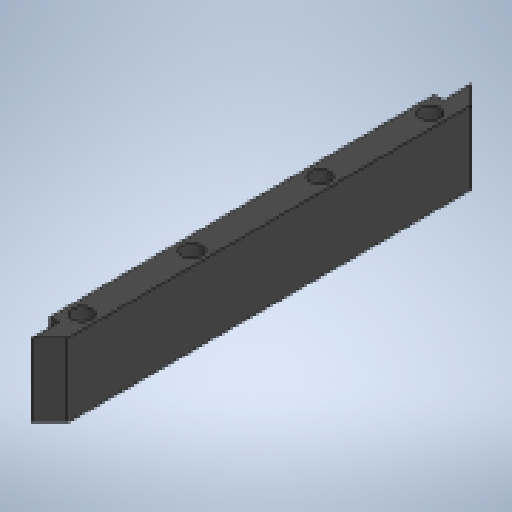
# Autodesk Inventor part: Backplate
Saved by Autodesk Inventor 2023.2 (Build 272271000, 271)
## iProperties
Created: 2023-06-29
Part Number: Backplate
Material: UHMW, Black
Document SubType Name: Modeling
Designer: Nathan Cai
Density: 0.94 g/cm^3
Appearance: Rubber - Black
Author: Nathan Cai
Autodesk Inventor part; units mm, degrees
ref_plane "YZ Plane" through (0, 0, 0) normal (1, 0, 0) x (0, 1, 0)
ref_plane "XZ Plane" through (0, 0, 0) normal (0, 1, 0) x (-1, 0, 0)
ref_plane "XY Plane" through (0, 0, 0) normal (0, 0, 1) x (1, 0, 0)
sketch "Sketch1" plane through (0, 0, 0) normal (0, 1, 0) x (-1, 0, 0)
  line L0 (-4.7625, 66.675) -> (4.7625, 66.675)
  line L1 (4.7625, 66.675) -> (4.7625, -66.675)
  line L2 (4.7625, -66.675) -> (-4.7625, -66.675)
  line L3 (-4.7625, -66.675) -> (-4.7625, 66.675)
  line L4 (-4.7625, 66.675) -> (4.7625, -66.675) construction
  line L5 (4.7625, 66.675) -> (-4.7625, -66.675) construction
  line L6 (-4.7625, 66.675) -> (1.5875, 66.675)
  line L7 (1.5875, 66.675) -> (1.5875, 76.2)
  line L8 (1.5875, 76.2) -> (-4.7625, 76.2)
  line L9 (-4.7625, 76.2) -> (-4.7625, 66.675)
  line L10 (4.7625, 0) -> (-4.7625, 0) construction
  line L11 (-4.7625, -66.675) -> (1.5875, -66.675)
  line L12 (1.5875, -66.675) -> (1.5875, -76.2)
  line L13 (1.5875, -76.2) -> (-4.7625, -76.2)
  line L14 (-4.7625, -76.2) -> (-4.7625, -66.675)
  line L15 (0, 66.675) -> (0, -66.675) construction
  circle A0 centre (0, 60.325) radius 3.302
  circle A1 centre (0, 22.225) radius 3.302
  circle A2 centre (0, -60.325) radius 3.302
  circle A3 centre (0, -22.225) radius 3.302
  point P0 (0, 0)
  point P1 (0, 0)
  dimension "d0" = 9.525
  dimension "d1" = 133.35
  dimension "d2" = 6.35
  dimension "d3" = 9.525
  dimension "d4" = 6.604
  dimension "d5" = 6.35
  dimension "d6" = 6.604
  dimension "d7" = 22.225
  constraints: 32 end point, 6 midpoint, 5 symmetric about line, 4 centre point, 4 parallel, 4 point on line, 3 perpendicular, 2 horizontal, 2 other
  measures "d0" distance of L1.end L2.end
  measures "d1" distance of L0.end L1.end
  measures "d2" distance of L8.end L7.end
  measures "d3" distance of L7.end L6.end
  measures "d4" diameter of A0
  measures "d5" distance from line of L6 A0.centre
  measures "d6" diameter of A1
  measures "d7" distance from line of L10 A1.centre
extrude "Extrusion1" add sketch "Sketch1" along normal blind 25.4
chamfer "Chamfer1" distance 6.35 angle 45 2 edges at (4.7625, 12.7, 76.2) (4.7625, 12.7, -76.2)
body "Solid1"
